Autodesk Inventor part; units mm, degrees
(part 2 of 13)
  line L469 (36.754, 19.2324) -> (36.3194, 18.7979) construction
  line L470 (36.3194, 18.7979) -> (36.3194, 18.2619) construction
  spline S154 degree 3 poles (36.3194, 18.2619) (36.3194, 17.7259) (36.754, 17.2914) (37.29, 17.2914) knots 0 0 0 0 1 1 1 1
  line L471 (36.3194, 18.2619) -> (36.3194, 17.7259) construction
  line L472 (36.3194, 17.7259) -> (36.754, 17.2914) construction
  line L473 (36.754, 17.2914) -> (37.29, 17.2914) construction
  spline S155 degree 3 poles (37.29, 17.2914) (37.826, 17.2914) (38.2606, 17.7259) (38.2606, 18.2619) knots 0 0 0 0 1 1 1 1
  line L474 (37.29, 17.2914) -> (37.826, 17.2914) construction
  line L475 (37.826, 17.2914) -> (38.2606, 17.7259) construction
  line L476 (38.2606, 17.7259) -> (38.2606, 18.2619) construction
  spline S156 degree 3 poles (35.7064, 20.816) (35.7064, 21.352) (35.2719, 21.7866) (34.7358, 21.7866) knots 0 0 0 0 1 1 1 1
  line L477 (35.7064, 20.816) -> (35.7064, 21.352) construction
  line L478 (35.7064, 21.352) -> (35.2719, 21.7866) construction
  line L479 (35.2719, 21.7866) -> (34.7358, 21.7866) construction
  spline S157 degree 3 poles (34.7358, 21.7866) (34.1999, 21.7866) (33.7653, 21.352) (33.7653, 20.816) knots 0 0 0 0 1 1 1 1
  line L480 (34.7358, 21.7866) -> (34.1999, 21.7866) construction
  line L481 (34.1999, 21.7866) -> (33.7653, 21.352) construction
  line L482 (33.7653, 21.352) -> (33.7653, 20.816) construction
  spline S158 degree 3 poles (33.7653, 20.816) (33.7653, 20.28) (34.1999, 19.8455) (34.7358, 19.8455) knots 0 0 0 0 1 1 1 1
  line L483 (33.7653, 20.816) -> (33.7653, 20.28) construction
  line L484 (33.7653, 20.28) -> (34.1999, 19.8455) construction
  line L485 (34.1999, 19.8455) -> (34.7358, 19.8455) construction
  spline S159 degree 3 poles (34.7358, 19.8455) (35.2719, 19.8455) (35.7064, 20.28) (35.7064, 20.816) knots 0 0 0 0 1 1 1 1
  line L486 (34.7358, 19.8455) -> (35.2719, 19.8455) construction
  line L487 (35.2719, 19.8455) -> (35.7064, 20.28) construction
  line L488 (35.7064, 20.28) -> (35.7064, 20.816) construction
  spline S160 degree 3 poles (35.7064, 23.3701) (35.7064, 23.9061) (35.2719, 24.3407) (34.7358, 24.3407) knots 0 0 0 0 1 1 1 1
  line L489 (35.7064, 23.3701) -> (35.7064, 23.9061) construction
  line L490 (35.7064, 23.9061) -> (35.2719, 24.3407) construction
  line L491 (35.2719, 24.3407) -> (34.7358, 24.3407) construction
  spline S161 degree 3 poles (34.7358, 24.3407) (34.1999, 24.3407) (33.7653, 23.9061) (33.7653, 23.3701) knots 0 0 0 0 1 1 1 1
  line L492 (34.7358, 24.3407) -> (34.1999, 24.3407) construction
  line L493 (34.1999, 24.3407) -> (33.7653, 23.9061) construction
  line L494 (33.7653, 23.9061) -> (33.7653, 23.3701) construction
  spline S162 degree 3 poles (33.7653, 23.3701) (33.7653, 22.8341) (34.1999, 22.3996) (34.7358, 22.3996) knots 0 0 0 0 1 1 1 1
  line L495 (33.7653, 23.3701) -> (33.7653, 22.8341) construction
  line L496 (33.7653, 22.8341) -> (34.1999, 22.3996) construction
  line L497 (34.1999, 22.3996) -> (34.7358, 22.3996) construction
  spline S163 degree 3 poles (34.7358, 22.3996) (35.2719, 22.3996) (35.7064, 22.8341) (35.7064, 23.3701) knots 0 0 0 0 1 1 1 1
  line L498 (34.7358, 22.3996) -> (35.2719, 22.3996) construction
  line L499 (35.2719, 22.3996) -> (35.7064, 22.8341) construction
  line L500 (35.7064, 22.8341) -> (35.7064, 23.3701) construction
  spline S164 degree 3 poles (35.7064, 25.9242) (35.7064, 26.4602) (35.2719, 26.8948) (34.7358, 26.8948) knots 0 0 0 0 1 1 1 1
  line L501 (35.7064, 25.9242) -> (35.7064, 26.4602) construction
  line L502 (35.7064, 26.4602) -> (35.2719, 26.8948) construction
  line L503 (35.2719, 26.8948) -> (34.7358, 26.8948) construction
  spline S165 degree 3 poles (34.7358, 26.8948) (34.1999, 26.8948) (33.7653, 26.4602) (33.7653, 25.9242) knots 0 0 0 0 1 1 1 1
  line L504 (34.7358, 26.8948) -> (34.1999, 26.8948) construction
  line L505 (34.1999, 26.8948) -> (33.7653, 26.4602) construction
  line L506 (33.7653, 26.4602) -> (33.7653, 25.9242) construction
  spline S166 degree 3 poles (33.7653, 25.9242) (33.7653, 25.3882) (34.1999, 24.9537) (34.7358, 24.9537) knots 0 0 0 0 1 1 1 1
  line L507 (33.7653, 25.9242) -> (33.7653, 25.3882) construction
  line L508 (33.7653, 25.3882) -> (34.1999, 24.9537) construction
  line L509 (34.1999, 24.9537) -> (34.7358, 24.9537) construction
  spline S167 degree 3 poles (34.7358, 24.9537) (35.2719, 24.9537) (35.7064, 25.3882) (35.7064, 25.9242) knots 0 0 0 0 1 1 1 1
  line L510 (34.7358, 24.9537) -> (35.2719, 24.9537) construction
  line L511 (35.2719, 24.9537) -> (35.7064, 25.3882) construction
  line L512 (35.7064, 25.3882) -> (35.7064, 25.9242) construction
  spline S168 degree 3 poles (35.7064, 28.4784) (35.7064, 29.0143) (35.2719, 29.4489) (34.7358, 29.4489) knots 0 0 0 0 1 1 1 1
  line L513 (35.7064, 28.4784) -> (35.7064, 29.0143) construction
  line L514 (35.7064, 29.0143) -> (35.2719, 29.4489) construction
  line L515 (35.2719, 29.4489) -> (34.7358, 29.4489) construction
  spline S169 degree 3 poles (34.7358, 29.4489) (34.1999, 29.4489) (33.7653, 29.0143) (33.7653, 28.4784) knots 0 0 0 0 1 1 1 1
  line L516 (34.7358, 29.4489) -> (34.1999, 29.4489) construction
  line L517 (34.1999, 29.4489) -> (33.7653, 29.0143) construction
  line L518 (33.7653, 29.0143) -> (33.7653, 28.4784) construction
  spline S170 degree 3 poles (33.7653, 28.4784) (33.7653, 27.9423) (34.1999, 27.5078) (34.7358, 27.5078) knots 0 0 0 0 1 1 1 1
  line L519 (33.7653, 28.4784) -> (33.7653, 27.9423) construction
  line L520 (33.7653, 27.9423) -> (34.1999, 27.5078) construction
  line L521 (34.1999, 27.5078) -> (34.7358, 27.5078) construction
  spline S171 degree 3 poles (34.7358, 27.5078) (35.2719, 27.5078) (35.7064, 27.9423) (35.7064, 28.4784) knots 0 0 0 0 1 1 1 1
  line L522 (34.7358, 27.5078) -> (35.2719, 27.5078) construction
  line L523 (35.2719, 27.5078) -> (35.7064, 27.9423) construction
  line L524 (35.7064, 27.9423) -> (35.7064, 28.4784) construction
  spline S172 degree 3 poles (35.7064, 31.0325) (35.7064, 31.5684) (35.2719, 32.003) (34.7358, 32.003) knots 0 0 0 0 1 1 1 1
  line L525 (35.7064, 31.0325) -> (35.7064, 31.5684) construction
  line L526 (35.7064, 31.5684) -> (35.2719, 32.003) construction
  line L527 (35.2719, 32.003) -> (34.7358, 32.003) construction
  spline S173 degree 3 poles (34.7358, 32.003) (34.1999, 32.003) (33.7653, 31.5684) (33.7653, 31.0325) knots 0 0 0 0 1 1 1 1
  line L528 (34.7358, 32.003) -> (34.1999, 32.003) construction
  line L529 (34.1999, 32.003) -> (33.7653, 31.5684) construction
  line L530 (33.7653, 31.5684) -> (33.7653, 31.0325) construction
  spline S174 degree 3 poles (33.7653, 31.0325) (33.7653, 30.4965) (34.1999, 30.0619) (34.7358, 30.0619) knots 0 0 0 0 1 1 1 1
  line L531 (33.7653, 31.0325) -> (33.7653, 30.4965) construction
  line L532 (33.7653, 30.4965) -> (34.1999, 30.0619) construction
  line L533 (34.1999, 30.0619) -> (34.7358, 30.0619) construction
  spline S175 degree 3 poles (34.7358, 30.0619) (35.2719, 30.0619) (35.7064, 30.4965) (35.7064, 31.0325) knots 0 0 0 0 1 1 1 1
  line L534 (34.7358, 30.0619) -> (35.2719, 30.0619) construction
  line L535 (35.2719, 30.0619) -> (35.7064, 30.4965) construction
  line L536 (35.7064, 30.4965) -> (35.7064, 31.0325) construction
  spline S176 degree 3 poles (38.2606, 20.816) (38.2606, 21.352) (37.826, 21.7866) (37.29, 21.7866) knots 0 0 0 0 1 1 1 1
  line L537 (38.2606, 20.816) -> (38.2606, 21.352) construction
  line L538 (38.2606, 21.352) -> (37.826, 21.7866) construction
  line L539 (37.826, 21.7866) -> (37.29, 21.7866) construction
  spline S177 degree 3 poles (37.29, 21.7866) (36.754, 21.7866) (36.3194, 21.352) (36.3194, 20.816) knots 0 0 0 0 1 1 1 1
  line L540 (37.29, 21.7866) -> (36.754, 21.7866) construction
  line L541 (36.754, 21.7866) -> (36.3194, 21.352) construction
  line L542 (36.3194, 21.352) -> (36.3194, 20.816) construction
  spline S178 degree 3 poles (36.3194, 20.816) (36.3194, 20.28) (36.754, 19.8455) (37.29, 19.8455) knots 0 0 0 0 1 1 1 1
  line L543 (36.3194, 20.816) -> (36.3194, 20.28) construction
  line L544 (36.3194, 20.28) -> (36.754, 19.8455) construction
  line L545 (36.754, 19.8455) -> (37.29, 19.8455) construction
  spline S179 degree 3 poles (37.29, 19.8455) (37.826, 19.8455) (38.2606, 20.28) (38.2606, 20.816) knots 0 0 0 0 1 1 1 1
  line L546 (37.29, 19.8455) -> (37.826, 19.8455) construction
  line L547 (37.826, 19.8455) -> (38.2606, 20.28) construction
  line L548 (38.2606, 20.28) -> (38.2606, 20.816) construction
  spline S180 degree 3 poles (38.2606, 23.3701) (38.2606, 23.9061) (37.826, 24.3407) (37.29, 24.3407) knots 0 0 0 0 1 1 1 1
  line L549 (38.2606, 23.3701) -> (38.2606, 23.9061) construction
  line L550 (38.2606, 23.9061) -> (37.826, 24.3407) construction
  line L551 (37.826, 24.3407) -> (37.29, 24.3407) construction
  spline S181 degree 3 poles (37.29, 24.3407) (36.754, 24.3407) (36.3194, 23.9061) (36.3194, 23.3701) knots 0 0 0 0 1 1 1 1
  line L552 (37.29, 24.3407) -> (36.754, 24.3407) construction
  line L553 (36.754, 24.3407) -> (36.3194, 23.9061) construction
  line L554 (36.3194, 23.9061) -> (36.3194, 23.3701) construction
  spline S182 degree 3 poles (36.3194, 23.3701) (36.3194, 22.8341) (36.754, 22.3996) (37.29, 22.3996) knots 0 0 0 0 1 1 1 1
  line L555 (36.3194, 23.3701) -> (36.3194, 22.8341) construction
  line L556 (36.3194, 22.8341) -> (36.754, 22.3996) construction
  line L557 (36.754, 22.3996) -> (37.29, 22.3996) construction
  spline S183 degree 3 poles (37.29, 22.3996) (37.826, 22.3996) (38.2606, 22.8341) (38.2606, 23.3701) knots 0 0 0 0 1 1 1 1
  line L558 (37.29, 22.3996) -> (37.826, 22.3996) construction
  line L559 (37.826, 22.3996) -> (38.2606, 22.8341) construction
  line L560 (38.2606, 22.8341) -> (38.2606, 23.3701) construction
  spline S184 degree 3 poles (38.2606, 25.9242) (38.2606, 26.4602) (37.826, 26.8948) (37.29, 26.8948) knots 0 0 0 0 1 1 1 1
  line L561 (38.2606, 25.9242) -> (38.2606, 26.4602) construction
  line L562 (38.2606, 26.4602) -> (37.826, 26.8948) construction
  line L563 (37.826, 26.8948) -> (37.29, 26.8948) construction
  spline S185 degree 3 poles (37.29, 26.8948) (36.754, 26.8948) (36.3194, 26.4602) (36.3194, 25.9242) knots 0 0 0 0 1 1 1 1
  line L564 (37.29, 26.8948) -> (36.754, 26.8948) construction
  line L565 (36.754, 26.8948) -> (36.3194, 26.4602) construction
  line L566 (36.3194, 26.4602) -> (36.3194, 25.9242) construction
  spline S186 degree 3 poles (36.3194, 25.9242) (36.3194, 25.3882) (36.754, 24.9537) (37.29, 24.9537) knots 0 0 0 0 1 1 1 1
  line L567 (36.3194, 25.9242) -> (36.3194, 25.3882) construction
  line L568 (36.3194, 25.3882) -> (36.754, 24.9537) construction
  line L569 (36.754, 24.9537) -> (37.29, 24.9537) construction
  spline S187 degree 3 poles (37.29, 24.9537) (37.826, 24.9537) (38.2606, 25.3882) (38.2606, 25.9242) knots 0 0 0 0 1 1 1 1
  line L570 (37.29, 24.9537) -> (37.826, 24.9537) construction
  line L571 (37.826, 24.9537) -> (38.2606, 25.3882) construction
  line L572 (38.2606, 25.3882) -> (38.2606, 25.9242) construction
  spline S188 degree 3 poles (38.2606, 28.4784) (38.2606, 29.0143) (37.826, 29.4489) (37.29, 29.4489) knots 0 0 0 0 1 1 1 1
  line L573 (38.2606, 28.4784) -> (38.2606, 29.0143) construction
  line L574 (38.2606, 29.0143) -> (37.826, 29.4489) construction
  line L575 (37.826, 29.4489) -> (37.29, 29.4489) construction
  spline S189 degree 3 poles (37.29, 29.4489) (36.754, 29.4489) (36.3194, 29.0143) (36.3194, 28.4784) knots 0 0 0 0 1 1 1 1
  line L576 (37.29, 29.4489) -> (36.754, 29.4489) construction
  line L577 (36.754, 29.4489) -> (36.3194, 29.0143) construction
  line L578 (36.3194, 29.0143) -> (36.3194, 28.4784) construction
  spline S190 degree 3 poles (36.3194, 28.4784) (36.3194, 27.9423) (36.754, 27.5078) (37.29, 27.5078) knots 0 0 0 0 1 1 1 1
  line L579 (36.3194, 28.4784) -> (36.3194, 27.9423) construction
  line L580 (36.3194, 27.9423) -> (36.754, 27.5078) construction
  line L581 (36.754, 27.5078) -> (37.29, 27.5078) construction
  spline S191 degree 3 poles (37.29, 27.5078) (37.826, 27.5078) (38.2606, 27.9423) (38.2606, 28.4784) knots 0 0 0 0 1 1 1 1
  line L582 (37.29, 27.5078) -> (37.826, 27.5078) construction
  line L583 (37.826, 27.5078) -> (38.2606, 27.9423) construction
  line L584 (38.2606, 27.9423) -> (38.2606, 28.4784) construction
  spline S192 degree 3 poles (38.2606, 31.0325) (38.2606, 31.5684) (37.826, 32.003) (37.29, 32.003) knots 0 0 0 0 1 1 1 1
  line L585 (38.2606, 31.0325) -> (38.2606, 31.5684) construction
  line L586 (38.2606, 31.5684) -> (37.826, 32.003) construction
  line L587 (37.826, 32.003) -> (37.29, 32.003) construction
  spline S193 degree 3 poles (37.29, 32.003) (36.754, 32.003) (36.3194, 31.5684) (36.3194, 31.0325) knots 0 0 0 0 1 1 1 1
  line L588 (37.29, 32.003) -> (36.754, 32.003) construction
  line L589 (36.754, 32.003) -> (36.3194, 31.5684) construction
  line L590 (36.3194, 31.5684) -> (36.3194, 31.0325) construction
  spline S194 degree 3 poles (36.3194, 31.0325) (36.3194, 30.4965) (36.754, 30.0619) (37.29, 30.0619) knots 0 0 0 0 1 1 1 1
  line L591 (36.3194, 31.0325) -> (36.3194, 30.4965) construction
  line L592 (36.3194, 30.4965) -> (36.754, 30.0619) construction
  line L593 (36.754, 30.0619) -> (37.29, 30.0619) construction
  spline S195 degree 3 poles (37.29, 30.0619) (37.826, 30.0619) (38.2606, 30.4965) (38.2606, 31.0325) knots 0 0 0 0 1 1 1 1
  line L594 (37.29, 30.0619) -> (37.826, 30.0619) construction
  line L595 (37.826, 30.0619) -> (38.2606, 30.4965) construction
  line L596 (38.2606, 30.4965) -> (38.2606, 31.0325) construction
  spline S196 degree 3 poles (45.9229, 0.3832) (45.9229, 0.9191) (45.4883, 1.3537) (44.9523, 1.3537) knots 0 0 0 0 1 1 1 1
  line L597 (45.9229, 0.3832) -> (45.9229, 0.9191) construction
  line L598 (45.9229, 0.9191) -> (45.4883, 1.3537) construction
  line L599 (45.4883, 1.3537) -> (44.9523, 1.3537) construction
  spline S197 degree 3 poles (44.9523, 1.3537) (44.4163, 1.3537) (43.9818, 0.9191) (43.9818, 0.3832) knots 0 0 0 0 1 1 1 1
  line L600 (44.9523, 1.3537) -> (44.4163, 1.3537) construction
  line L601 (44.4163, 1.3537) -> (43.9818, 0.9191) construction
  line L602 (43.9818, 0.9191) -> (43.9818, 0.3832) construction
  spline S198 degree 3 poles (43.9818, 0.3832) (43.9818, -0.1529) (44.4163, -0.5874) (44.9523, -0.5874) knots 0 0 0 0 1 1 1 1
  line L603 (43.9818, 0.3832) -> (43.9818, -0.1529) construction
  line L604 (43.9818, -0.1529) -> (44.4163, -0.5874) construction
  line L605 (44.4163, -0.5874) -> (44.9523, -0.5874) construction
  spline S199 degree 3 poles (44.9523, -0.5874) (45.4883, -0.5874) (45.9229, -0.1529) (45.9229, 0.3832) knots 0 0 0 0 1 1 1 1
  line L606 (44.9523, -0.5874) -> (45.4883, -0.5874) construction
  line L607 (45.4883, -0.5874) -> (45.9229, -0.1529) construction
  line L608 (45.9229, -0.1529) -> (45.9229, 0.3832) construction
  spline S200 degree 3 poles (48.477, 0.3832) (48.477, 0.9191) (48.0424, 1.3537) (47.5064, 1.3537) knots 0 0 0 0 1 1 1 1
  line L609 (48.477, 0.3832) -> (48.477, 0.9191) construction
  line L610 (48.477, 0.9191) -> (48.0424, 1.3537) construction
  line L611 (48.0424, 1.3537) -> (47.5064, 1.3537) construction
  spline S201 degree 3 poles (47.5064, 1.3537) (46.9704, 1.3537) (46.5359, 0.9191) (46.5359, 0.3832) knots 0 0 0 0 1 1 1 1
  line L612 (47.5064, 1.3537) -> (46.9704, 1.3537) construction
  line L613 (46.9704, 1.3537) -> (46.5359, 0.9191) construction
  line L614 (46.5359, 0.9191) -> (46.5359, 0.3832) construction
  spline S202 degree 3 poles (46.5359, 0.3832) (46.5359, -0.1529) (46.9704, -0.5874) (47.5064, -0.5874) knots 0 0 0 0 1 1 1 1
  line L615 (46.5359, 0.3832) -> (46.5359, -0.1529) construction
  line L616 (46.5359, -0.1529) -> (46.9704, -0.5874) construction
  line L617 (46.9704, -0.5874) -> (47.5064, -0.5874) construction
  spline S203 degree 3 poles (47.5064, -0.5874) (48.0424, -0.5874) (48.477, -0.1529) (48.477, 0.3832) knots 0 0 0 0 1 1 1 1
  line L618 (47.5064, -0.5874) -> (48.0424, -0.5874) construction
  line L619 (48.0424, -0.5874) -> (48.477, -0.1529) construction
  line L620 (48.477, -0.1529) -> (48.477, 0.3832) construction
  spline S204 degree 3 poles (47.3149, 9.7057) (47.3149, 10.9399) (46.3142, 11.9405) (45.08, 11.9405) knots 0 0 0 0 1 1 1 1
  line L621 (47.3149, 9.7057) -> (47.3149, 10.9399) construction
  line L622 (47.3149, 10.9399) -> (46.3142, 11.9405) construction
  line L623 (46.3142, 11.9405) -> (45.08, 11.9405) construction
  spline S205 degree 3 poles (45.08, 11.9405) (43.8459, 11.9405) (42.8452, 10.9399) (42.8452, 9.7057) knots 0 0 0 0 1 1 1 1
  line L624 (45.08, 11.9405) -> (43.8459, 11.9405) construction
  line L625 (43.8459, 11.9405) -> (42.8452, 10.9399) construction
  line L626 (42.8452, 10.9399) -> (42.8452, 9.7057) construction
  spline S206 degree 3 poles (42.8452, 9.7057) (42.8452, 8.4714) (43.8459, 7.4708) (45.08, 7.4708) knots 0 0 0 0 1 1 1 1
  line L627 (42.8452, 9.7057) -> (42.8452, 8.4714) construction
  line L628 (42.8452, 8.4714) -> (43.8459, 7.4708) construction
  line L629 (43.8459, 7.4708) -> (45.08, 7.4708) construction
  spline S207 degree 3 poles (45.08, 7.4708) (46.3142, 7.4708) (47.3149, 8.4714) (47.3149, 9.7057) knots 0 0 0 0 1 1 1 1
  line L630 (45.08, 7.4708) -> (46.3142, 7.4708) construction
  line L631 (46.3142, 7.4708) -> (47.3149, 8.4714) construction
  line L632 (47.3149, 8.4714) -> (47.3149, 9.7057) construction
  spline S208 degree 3 poles (53.5724, 9.7057) (53.5724, 10.8694) (52.6292, 11.8128) (51.4653, 11.8128) knots 0 0 0 0 1 1 1 1
  line L633 (53.5724, 9.7057) -> (53.5724, 10.8694) construction
  line L634 (53.5724, 10.8694) -> (52.6292, 11.8128) construction
  line L635 (52.6292, 11.8128) -> (51.4653, 11.8128) construction
  spline S209 degree 3 poles (51.4653, 11.8128) (50.3018, 11.8128) (49.3582, 10.8694) (49.3582, 9.7057) knots 0 0 0 0 1 1 1 1
  line L636 (51.4653, 11.8128) -> (50.3018, 11.8128) construction
  line L637 (50.3018, 11.8128) -> (49.3582, 10.8694) construction
  line L638 (49.3582, 10.8694) -> (49.3582, 9.7057) construction
  spline S210 degree 3 poles (49.3582, 9.7057) (49.3582, 8.542) (50.3018, 7.5984) (51.4653, 7.5984) knots 0 0 0 0 1 1 1 1
  line L639 (49.3582, 9.7057) -> (49.3582, 8.542) construction
  line L640 (49.3582, 8.542) -> (50.3018, 7.5984) construction
  line L641 (50.3018, 7.5984) -> (51.4653, 7.5984) construction
  spline S211 degree 3 poles (51.4653, 7.5984) (52.6292, 7.5984) (53.5724, 8.542) (53.5724, 9.7057) knots 0 0 0 0 1 1 1 1
  line L642 (51.4653, 7.5984) -> (52.6292, 7.5984) construction
  line L643 (52.6292, 7.5984) -> (53.5724, 8.542) construction
  line L644 (53.5724, 8.542) -> (53.5724, 9.7057) construction
  spline S212 degree 3 poles (50.316, 14.303) (50.316, 15.4314) (49.4011, 16.3463) (48.2727, 16.3463) knots 0 0 0 0 1 1 1 1
  line L645 (50.316, 14.303) -> (50.316, 15.4314) construction
  line L646 (50.316, 15.4314) -> (49.4011, 16.3463) construction
  line L647 (49.4011, 16.3463) -> (48.2727, 16.3463) construction
  spline S213 degree 3 poles (48.2727, 16.3463) (47.1442, 16.3463) (46.2294, 15.4314) (46.2294, 14.303) knots 0 0 0 0 1 1 1 1
  line L648 (48.2727, 16.3463) -> (47.1442, 16.3463) construction
  line L649 (47.1442, 16.3463) -> (46.2294, 15.4314) construction
  line L650 (46.2294, 15.4314) -> (46.2294, 14.303) construction
  spline S214 degree 3 poles (46.2294, 14.303) (46.2294, 13.1746) (47.1442, 12.2598) (48.2727, 12.2598) knots 0 0 0 0 1 1 1 1
  line L651 (46.2294, 14.303) -> (46.2294, 13.1746) construction
  line L652 (46.2294, 13.1746) -> (47.1442, 12.2598) construction
  line L653 (47.1442, 12.2598) -> (48.2727, 12.2598) construction
  spline S215 degree 3 poles (48.2727, 12.2598) (49.4011, 12.2598) (50.316, 13.1746) (50.316, 14.303) knots 0 0 0 0 1 1 1 1
  line L654 (48.2727, 12.2598) -> (49.4011, 12.2598) construction
  line L655 (49.4011, 12.2598) -> (50.316, 13.1746) construction
  line L656 (50.316, 13.1746) -> (50.316, 14.303) construction
  spline S216 degree 3 poles (10.1653, 0.3832) (10.1653, 0.9191) (9.7308, 1.3537) (9.1948, 1.3537) knots 0 0 0 0 1 1 1 1
  line L657 (10.1653, 0.3832) -> (10.1653, 0.9191) construction
  line L658 (10.1653, 0.9191) -> (9.7308, 1.3537) construction
  line L659 (9.7308, 1.3537) -> (9.1948, 1.3537) construction
  spline S217 degree 3 poles (9.1948, 1.3537) (8.6588, 1.3537) (8.2242, 0.9191) (8.2242, 0.3832) knots 0 0 0 0 1 1 1 1
  line L660 (9.1948, 1.3537) -> (8.6588, 1.3537) construction
  line L661 (8.6588, 1.3537) -> (8.2242, 0.9191) construction
  line L662 (8.2242, 0.9191) -> (8.2242, 0.3832) construction
  spline S218 degree 3 poles (8.2242, 0.3832) (8.2242, -0.1529) (8.6588, -0.5874) (9.1948, -0.5874) knots 0 0 0 0 1 1 1 1
  line L663 (8.2242, 0.3832) -> (8.2242, -0.1529) construction
  line L664 (8.2242, -0.1529) -> (8.6588, -0.5874) construction
  line L665 (8.6588, -0.5874) -> (9.1948, -0.5874) construction
  spline S219 degree 3 poles (9.1948, -0.5874) (9.7308, -0.5874) (10.1653, -0.1529) (10.1653, 0.3832) knots 0 0 0 0 1 1 1 1
  line L666 (9.1948, -0.5874) -> (9.7308, -0.5874) construction
  line L667 (9.7308, -0.5874) -> (10.1653, -0.1529) construction
  line L668 (10.1653, -0.1529) -> (10.1653, 0.3832) construction
  spline S220 degree 3 poles (12.7194, 0.3832) (12.7194, 0.9191) (12.2849, 1.3537) (11.7489, 1.3537) knots 0 0 0 0 1 1 1 1
  line L669 (12.7194, 0.3832) -> (12.7194, 0.9191) construction
  line L670 (12.7194, 0.9191) -> (12.2849, 1.3537) construction
  line L671 (12.2849, 1.3537) -> (11.7489, 1.3537) construction
  spline S221 degree 3 poles (11.7489, 1.3537) (11.2129, 1.3537) (10.7783, 0.9191) (10.7783, 0.3832) knots 0 0 0 0 1 1 1 1
  line L672 (11.7489, 1.3537) -> (11.2129, 1.3537) construction
  line L673 (11.2129, 1.3537) -> (10.7783, 0.9191) construction
  line L674 (10.7783, 0.9191) -> (10.7783, 0.3832) construction
  spline S222 degree 3 poles (10.7783, 0.3832) (10.7783, -0.1529) (11.2129, -0.5874) (11.7489, -0.5874) knots 0 0 0 0 1 1 1 1
  line L675 (10.7783, 0.3832) -> (10.7783, -0.1529) construction
  line L676 (10.7783, -0.1529) -> (11.2129, -0.5874) construction
  line L677 (11.2129, -0.5874) -> (11.7489, -0.5874) construction
  spline S223 degree 3 poles (11.7489, -0.5874) (12.2849, -0.5874) (12.7194, -0.1529) (12.7194, 0.3832) knots 0 0 0 0 1 1 1 1
  line L678 (11.7489, -0.5874) -> (12.2849, -0.5874) construction
  line L679 (12.2849, -0.5874) -> (12.7194, -0.1529) construction
  line L680 (12.7194, -0.1529) -> (12.7194, 0.3832) construction
  spline S224 degree 3 poles (15.2735, 0.3832) (15.2735, 0.9191) (14.839, 1.3537) (14.303, 1.3537) knots 0 0 0 0 1 1 1 1
  line L681 (15.2735, 0.3832) -> (15.2735, 0.9191) construction
  line L682 (15.2735, 0.9191) -> (14.839, 1.3537) construction
  line L683 (14.839, 1.3537) -> (14.303, 1.3537) construction
  spline S225 degree 3 poles (14.303, 1.3537) (13.767, 1.3537) (13.3324, 0.9191) (13.3324, 0.3832) knots 0 0 0 0 1 1 1 1
  line L684 (14.303, 1.3537) -> (13.767, 1.3537) construction
  line L685 (13.767, 1.3537) -> (13.3324, 0.9191) construction
  line L686 (13.3324, 0.9191) -> (13.3324, 0.3832) construction
  spline S226 degree 3 poles (13.3324, 0.3832) (13.3324, -0.1529) (13.767, -0.5874) (14.303, -0.5874) knots 0 0 0 0 1 1 1 1
  line L687 (13.3324, 0.3832) -> (13.3324, -0.1529) construction
  line L688 (13.3324, -0.1529) -> (13.767, -0.5874) construction
  line L689 (13.767, -0.5874) -> (14.303, -0.5874) construction
  spline S227 degree 3 poles (14.303, -0.5874) (14.839, -0.5874) (15.2735, -0.1529) (15.2735, 0.3832) knots 0 0 0 0 1 1 1 1
  line L690 (14.303, -0.5874) -> (14.839, -0.5874) construction
  line L691 (14.839, -0.5874) -> (15.2735, -0.1529) construction
  line L692 (15.2735, -0.1529) -> (15.2735, 0.3832) construction
  spline S228 degree 3 poles (17.8276, 0.3832) (17.8276, 0.9191) (17.3931, 1.3537) (16.8571, 1.3537) knots 0 0 0 0 1 1 1 1
  line L693 (17.8276, 0.3832) -> (17.8276, 0.9191) construction
  line L694 (17.8276, 0.9191) -> (17.3931, 1.3537) construction
  line L695 (17.3931, 1.3537) -> (16.8571, 1.3537) construction
  spline S229 degree 3 poles (16.8571, 1.3537) (16.3211, 1.3537) (15.8866, 0.9191) (15.8866, 0.3832) knots 0 0 0 0 1 1 1 1
  line L696 (16.8571, 1.3537) -> (16.3211, 1.3537) construction
  line L697 (16.3211, 1.3537) -> (15.8866, 0.9191) construction
  line L698 (15.8866, 0.9191) -> (15.8866, 0.3832) construction
  spline S230 degree 3 poles (15.8866, 0.3832) (15.8866, -0.1529) (16.3211, -0.5874) (16.8571, -0.5874) knots 0 0 0 0 1 1 1 1
  line L699 (15.8866, 0.3832) -> (15.8866, -0.1529) construction
  line L700 (15.8866, -0.1529) -> (16.3211, -0.5874) construction
  line L701 (16.3211, -0.5874) -> (16.8571, -0.5874) construction
  spline S231 degree 3 poles (16.8571, -0.5874) (17.3931, -0.5874) (17.8276, -0.1529) (17.8276, 0.3832) knots 0 0 0 0 1 1 1 1
  line L702 (16.8571, -0.5874) -> (17.3931, -0.5874) construction
  line L703 (17.3931, -0.5874) -> (17.8276, -0.1529) construction
  line L704 (17.8276, -0.1529) -> (17.8276, 0.3832) construction
  spline S232 degree 3 poles (17.8276, 2.9373) (17.8276, 3.4732) (17.3931, 3.9078) (16.8571, 3.9078) knots 0 0 0 0 1 1 1 1
  line L705 (17.8276, 2.9373) -> (17.8276, 3.4732) construction
  line L706 (17.8276, 3.4732) -> (17.3931, 3.9078) construction
  line L707 (17.3931, 3.9078) -> (16.8571, 3.9078) construction
  spline S233 degree 3 poles (16.8571, 3.9078) (16.3211, 3.9078) (15.8866, 3.4732) (15.8866, 2.9373) knots 0 0 0 0 1 1 1 1
  line L708 (16.8571, 3.9078) -> (16.3211, 3.9078) construction
  line L709 (16.3211, 3.9078) -> (15.8866, 3.4732) construction
  line L710 (15.8866, 3.4732) -> (15.8866, 2.9373) construction
  spline S234 degree 3 poles (15.8866, 2.9373) (15.8866, 2.4013) (16.3211, 1.9667) (16.8571, 1.9667) knots 0 0 0 0 1 1 1 1
  line L711 (15.8866, 2.9373) -> (15.8866, 2.4013) construction
  line L712 (15.8866, 2.4013) -> (16.3211, 1.9667) construction
  line L713 (16.3211, 1.9667) -> (16.8571, 1.9667) construction
  spline S235 degree 3 poles (16.8571, 1.9667) (17.3931, 1.9667) (17.8276, 2.4013) (17.8276, 2.9373) knots 0 0 0 0 1 1 1 1
  line L714 (16.8571, 1.9667) -> (17.3931, 1.9667) construction
  line L715 (17.3931, 1.9667) -> (17.8276, 2.4013) construction
  line L716 (17.8276, 2.4013) -> (17.8276, 2.9373) construction
  spline S236 degree 3 poles (20.3818, 2.9373) (20.3818, 3.4732) (19.9472, 3.9078) (19.4112, 3.9078) knots 0 0 0 0 1 1 1 1
  line L717 (20.3818, 2.9373) -> (20.3818, 3.4732) construction
  line L718 (20.3818, 3.4732) -> (19.9472, 3.9078) construction
  line L719 (19.9472, 3.9078) -> (19.4112, 3.9078) construction
  spline S237 degree 3 poles (19.4112, 3.9078) (18.8752, 3.9078) (18.4407, 3.4732) (18.4407, 2.9373) knots 0 0 0 0 1 1 1 1
  line L720 (19.4112, 3.9078) -> (18.8752, 3.9078) construction
  line L721 (18.8752, 3.9078) -> (18.4407, 3.4732) construction
  line L722 (18.4407, 3.4732) -> (18.4407, 2.9373) construction
  spline S238 degree 3 poles (18.4407, 2.9373) (18.4407, 2.4013) (18.8752, 1.9667) (19.4112, 1.9667) knots 0 0 0 0 1 1 1 1
  line L723 (18.4407, 2.9373) -> (18.4407, 2.4013) construction
  line L724 (18.4407, 2.4013) -> (18.8752, 1.9667) construction
  line L725 (18.8752, 1.9667) -> (19.4112, 1.9667) construction
  spline S239 degree 3 poles (19.4112, 1.9667) (19.9472, 1.9667) (20.3818, 2.4013) (20.3818, 2.9373) knots 0 0 0 0 1 1 1 1
  line L726 (19.4112, 1.9667) -> (19.9472, 1.9667) construction
  line L727 (19.9472, 1.9667) -> (20.3818, 2.4013) construction
  line L728 (20.3818, 2.4013) -> (20.3818, 2.9373) construction
  spline S240 degree 3 poles (26.767, 0.3832) (26.767, 0.9191) (26.3325, 1.3537) (25.7965, 1.3537) knots 0 0 0 0 1 1 1 1
  line L729 (26.767, 0.3832) -> (26.767, 0.9191) construction
  line L730 (26.767, 0.9191) -> (26.3325, 1.3537) construction
  line L731 (26.3325, 1.3537) -> (25.7965, 1.3537) construction
  spline S241 degree 3 poles (25.7965, 1.3537) (25.2605, 1.3537) (24.8259, 0.9191) (24.8259, 0.3832) knots 0 0 0 0 1 1 1 1
  line L732 (25.7965, 1.3537) -> (25.2605, 1.3537) construction
  line L733 (25.2605, 1.3537) -> (24.8259, 0.9191) construction
  line L734 (24.8259, 0.9191) -> (24.8259, 0.3832) construction
  spline S242 degree 3 poles (24.8259, 0.3832) (24.8259, -0.1529) (25.2605, -0.5874) (25.7965, -0.5874) knots 0 0 0 0 1 1 1 1
  line L735 (24.8259, 0.3832) -> (24.8259, -0.1529) construction
  line L736 (24.8259, -0.1529) -> (25.2605, -0.5874) construction
  line L737 (25.2605, -0.5874) -> (25.7965, -0.5874) construction
  spline S243 degree 3 poles (25.7965, -0.5874) (26.3325, -0.5874) (26.767, -0.1529) (26.767, 0.3832) knots 0 0 0 0 1 1 1 1
  line L738 (25.7965, -0.5874) -> (26.3325, -0.5874) construction
  line L739 (26.3325, -0.5874) -> (26.767, -0.1529) construction
  line L740 (26.767, -0.1529) -> (26.767, 0.3832) construction
  spline S244 degree 3 poles (24.2129, 0.3832) (24.2129, 0.9191) (23.7784, 1.3537) (23.2424, 1.3537) knots 0 0 0 0 1 1 1 1
  line L741 (24.2129, 0.3832) -> (24.2129, 0.9191) construction
  line L742 (24.2129, 0.9191) -> (23.7784, 1.3537) construction
  line L743 (23.7784, 1.3537) -> (23.2424, 1.3537) construction
  spline S245 degree 3 poles (23.2424, 1.3537) (22.7064, 1.3537) (22.2718, 0.9191) (22.2718, 0.3832) knots 0 0 0 0 1 1 1 1
  line L744 (23.2424, 1.3537) -> (22.7064, 1.3537) construction
  line L745 (22.7064, 1.3537) -> (22.2718, 0.9191) construction
  line L746 (22.2718, 0.9191) -> (22.2718, 0.3832) construction
  spline S246 degree 3 poles (22.2718, 0.3832) (22.2718, -0.1529) (22.7064, -0.5874) (23.2424, -0.5874) knots 0 0 0 0 1 1 1 1
  line L747 (22.2718, 0.3832) -> (22.2718, -0.1529) construction
  line L748 (22.2718, -0.1529) -> (22.7064, -0.5874) construction
  line L749 (22.7064, -0.5874) -> (23.2424, -0.5874) construction
  spline S247 degree 3 poles (23.2424, -0.5874) (23.7784, -0.5874) (24.2129, -0.1529) (24.2129, 0.3832) knots 0 0 0 0 1 1 1 1
  line L750 (23.2424, -0.5874) -> (23.7784, -0.5874) construction
  line L751 (23.7784, -0.5874) -> (24.2129, -0.1529) construction
  line L752 (24.2129, -0.1529) -> (24.2129, 0.3832) construction
  spline S248 degree 3 poles (21.6588, 0.3832) (21.6588, 0.9191) (21.2243, 1.3537) (20.6882, 1.3537) knots 0 0 0 0 1 1 1 1
  line L753 (21.6588, 0.3832) -> (21.6588, 0.9191) construction
  line L754 (21.6588, 0.9191) -> (21.2243, 1.3537) construction
  line L755 (21.2243, 1.3537) -> (20.6882, 1.3537) construction
  spline S249 degree 3 poles (20.6882, 1.3537) (20.1523, 1.3537) (19.7177, 0.9191) (19.7177, 0.3832) knots 0 0 0 0 1 1 1 1
  line L756 (20.6882, 1.3537) -> (20.1523, 1.3537) construction
  line L757 (20.1523, 1.3537) -> (19.7177, 0.9191) construction
  line L758 (19.7177, 0.9191) -> (19.7177, 0.3832) construction
  spline S250 degree 3 poles (19.7177, 0.3832) (19.7177, -0.1529) (20.1523, -0.5874) (20.6882, -0.5874) knots 0 0 0 0 1 1 1 1
  line L759 (19.7177, 0.3832) -> (19.7177, -0.1529) construction
  line L760 (19.7177, -0.1529) -> (20.1523, -0.5874) construction
  line L761 (20.1523, -0.5874) -> (20.6882, -0.5874) construction
  spline S251 degree 3 poles (20.6882, -0.5874) (21.2243, -0.5874) (21.6588, -0.1529) (21.6588, 0.3832) knots 0 0 0 0 1 1 1 1
  line L762 (20.6882, -0.5874) -> (21.2243, -0.5874) construction
  line L763 (21.2243, -0.5874) -> (21.6588, -0.1529) construction
  line L764 (21.6588, -0.1529) -> (21.6588, 0.3832) construction
  spline S252 degree 3 poles (20.3818, 5.4914) (20.3818, 6.0273) (19.9472, 6.4619) (19.4112, 6.4619) knots 0 0 0 0 1 1 1 1
  line L765 (20.3818, 5.4914) -> (20.3818, 6.0273) construction
  line L766 (20.3818, 6.0273) -> (19.9472, 6.4619) construction
  line L767 (19.9472, 6.4619) -> (19.4112, 6.4619) construction
  spline S253 degree 3 poles (19.4112, 6.4619) (18.8752, 6.4619) (18.4407, 6.0273) (18.4407, 5.4914) knots 0 0 0 0 1 1 1 1
  line L768 (19.4112, 6.4619) -> (18.8752, 6.4619) construction
  line L769 (18.8752, 6.4619) -> (18.4407, 6.0273) construction
  line L770 (18.4407, 6.0273) -> (18.4407, 5.4914) construction
  spline S254 degree 3 poles (18.4407, 5.4914) (18.4407, 4.9554) (18.8752, 4.5208) (19.4112, 4.5208) knots 0 0 0 0 1 1 1 1
  line L771 (18.4407, 5.4914) -> (18.4407, 4.9554) construction
  line L772 (18.4407, 4.9554) -> (18.8752, 4.5208) construction
  line L773 (18.8752, 4.5208) -> (19.4112, 4.5208) construction
  spline S255 degree 3 poles (19.4112, 4.5208) (19.9472, 4.5208) (20.3818, 4.9554) (20.3818, 5.4914) knots 0 0 0 0 1 1 1 1
  line L774 (19.4112, 4.5208) -> (19.9472, 4.5208) construction
  line L775 (19.9472, 4.5208) -> (20.3818, 4.9554) construction
  line L776 (20.3818, 4.9554) -> (20.3818, 5.4914) construction
  spline S256 degree 3 poles (20.3818, 8.0455) (20.3818, 8.5815) (19.9472, 9.016) (19.4112, 9.016) knots 0 0 0 0 1 1 1 1
  line L777 (20.3818, 8.0455) -> (20.3818, 8.5815) construction
  line L778 (20.3818, 8.5815) -> (19.9472, 9.016) construction
  line L779 (19.9472, 9.016) -> (19.4112, 9.016) construction
  spline S257 degree 3 poles (19.4112, 9.016) (18.8752, 9.016) (18.4407, 8.5815) (18.4407, 8.0455) knots 0 0 0 0 1 1 1 1
  line L780 (19.4112, 9.016) -> (18.8752, 9.016) construction
  line L781 (18.8752, 9.016) -> (18.4407, 8.5815) construction
  line L782 (18.4407, 8.5815) -> (18.4407, 8.0455) construction
  spline S258 degree 3 poles (18.4407, 8.0455) (18.4407, 7.5095) (18.8752, 7.0749) (19.4112, 7.0749) knots 0 0 0 0 1 1 1 1
  line L783 (18.4407, 8.0455) -> (18.4407, 7.5095) construction
  line L784 (18.4407, 7.5095) -> (18.8752, 7.0749) construction
  line L785 (18.8752, 7.0749) -> (19.4112, 7.0749) construction
  spline S259 degree 3 poles (19.4112, 7.0749) (19.9472, 7.0749) (20.3818, 7.5095) (20.3818, 8.0455) knots 0 0 0 0 1 1 1 1
  line L786 (19.4112, 7.0749) -> (19.9472, 7.0749) construction
  line L787 (19.9472, 7.0749) -> (20.3818, 7.5095) construction
  line L788 (20.3818, 7.5095) -> (20.3818, 8.0455) construction
  spline S260 degree 3 poles (20.3818, 10.5996) (20.3818, 11.1356) (19.9472, 11.5701) (19.4112, 11.5701) knots 0 0 0 0 1 1 1 1
  line L789 (20.3818, 10.5996) -> (20.3818, 11.1356) construction
  line L790 (20.3818, 11.1356) -> (19.9472, 11.5701) construction
  line L791 (19.9472, 11.5701) -> (19.4112, 11.5701) construction
  spline S261 degree 3 poles (19.4112, 11.5701) (18.8752, 11.5701) (18.4407, 11.1356) (18.4407, 10.5996) knots 0 0 0 0 1 1 1 1
  line L792 (19.4112, 11.5701) -> (18.8752, 11.5701) construction
  line L793 (18.8752, 11.5701) -> (18.4407, 11.1356) construction
  line L794 (18.4407, 11.1356) -> (18.4407, 10.5996) construction
  spline S262 degree 3 poles (18.4407, 10.5996) (18.4407, 10.0636) (18.8752, 9.629) (19.4112, 9.629) knots 0 0 0 0 1 1 1 1
  line L795 (18.4407, 10.5996) -> (18.4407, 10.0636) construction
  line L796 (18.4407, 10.0636) -> (18.8752, 9.629) construction
  line L797 (18.8752, 9.629) -> (19.4112, 9.629) construction
  spline S263 degree 3 poles (19.4112, 9.629) (19.9472, 9.629) (20.3818, 10.0636) (20.3818, 10.5996) knots 0 0 0 0 1 1 1 1
  line L798 (19.4112, 9.629) -> (19.9472, 9.629) construction
  line L799 (19.9472, 9.629) -> (20.3818, 10.0636) construction
  line L800 (20.3818, 10.0636) -> (20.3818, 10.5996) construction
  spline S264 degree 3 poles (23.319, 11.7489) (23.319, 12.2849) (22.8844, 12.7194) (22.3485, 12.7194) knots 0 0 0 0 1 1 1 1
  line L801 (23.319, 11.7489) -> (23.319, 12.2849) construction
  line L802 (23.319, 12.2849) -> (22.8844, 12.7194) construction
  line L803 (22.8844, 12.7194) -> (22.3485, 12.7194) construction
  spline S265 degree 3 poles (22.3485, 12.7194) (21.8125, 12.7194) (21.3779, 12.2849) (21.3779, 11.7489) knots 0 0 0 0 1 1 1 1
  line L804 (22.3485, 12.7194) -> (21.8125, 12.7194) construction
  line L805 (21.8125, 12.7194) -> (21.3779, 12.2849) construction
  line L806 (21.3779, 12.2849) -> (21.3779, 11.7489) construction
  spline S266 degree 3 poles (21.3779, 11.7489) (21.3779, 11.2129) (21.8125, 10.7783) (22.3485, 10.7783) knots 0 0 0 0 1 1 1 1
  line L807 (21.3779, 11.7489) -> (21.3779, 11.2129) construction
  line L808 (21.3779, 11.2129) -> (21.8125, 10.7783) construction
  line L809 (21.8125, 10.7783) -> (22.3485, 10.7783) construction
  spline S267 degree 3 poles (22.3485, 10.7783) (22.8844, 10.7783) (23.319, 11.2129) (23.319, 11.7489) knots 0 0 0 0 1 1 1 1
  line L810 (22.3485, 10.7783) -> (22.8844, 10.7783) construction
  line L811 (22.8844, 10.7783) -> (23.319, 11.2129) construction
  line L812 (23.319, 11.2129) -> (23.319, 11.7489) construction
  spline S268 degree 3 poles (25.8731, 11.7489) (25.8731, 12.2849) (25.4385, 12.7194) (24.9026, 12.7194) knots 0 0 0 0 1 1 1 1
  line L813 (25.8731, 11.7489) -> (25.8731, 12.2849) construction
  line L814 (25.8731, 12.2849) -> (25.4385, 12.7194) construction
  line L815 (25.4385, 12.7194) -> (24.9026, 12.7194) construction
  spline S269 degree 3 poles (24.9026, 12.7194) (24.3666, 12.7194) (23.932, 12.2849) (23.932, 11.7489) knots 0 0 0 0 1 1 1 1
  line L816 (24.9026, 12.7194) -> (24.3666, 12.7194) construction
  line L817 (24.3666, 12.7194) -> (23.932, 12.2849) construction
  line L818 (23.932, 12.2849) -> (23.932, 11.7489) construction
  spline S270 degree 3 poles (23.932, 11.7489) (23.932, 11.2129) (24.3666, 10.7783) (24.9026, 10.7783) knots 0 0 0 0 1 1 1 1
  line L819 (23.932, 11.7489) -> (23.932, 11.2129) construction
  line L820 (23.932, 11.2129) -> (24.3666, 10.7783) construction
  line L821 (24.3666, 10.7783) -> (24.9026, 10.7783) construction
  spline S271 degree 3 poles (24.9026, 10.7783) (25.4385, 10.7783) (25.8731, 11.2129) (25.8731, 11.7489) knots 0 0 0 0 1 1 1 1
  line L822 (24.9026, 10.7783) -> (25.4385, 10.7783) construction
  line L823 (25.4385, 10.7783) -> (25.8731, 11.2129) construction
  line L824 (25.8731, 11.2129) -> (25.8731, 11.7489) construction
  spline S272 degree 3 poles (23.319, 14.303) (23.319, 14.839) (22.8844, 15.2735) (22.3485, 15.2735) knots 0 0 0 0 1 1 1 1
  line L825 (23.319, 14.303) -> (23.319, 14.839) construction
  line L826 (23.319, 14.839) -> (22.8844, 15.2735) construction
  line L827 (22.8844, 15.2735) -> (22.3485, 15.2735) construction
  spline S273 degree 3 poles (22.3485, 15.2735) (21.8125, 15.2735) (21.3779, 14.839) (21.3779, 14.303) knots 0 0 0 0 1 1 1 1
  line L828 (22.3485, 15.2735) -> (21.8125, 15.2735) construction
  line L829 (21.8125, 15.2735) -> (21.3779, 14.839) construction
  line L830 (21.3779, 14.839) -> (21.3779, 14.303) construction
  spline S274 degree 3 poles (21.3779, 14.303) (21.3779, 13.767) (21.8125, 13.3324) (22.3485, 13.3324) knots 0 0 0 0 1 1 1 1
  line L831 (21.3779, 14.303) -> (21.3779, 13.767) construction
  line L832 (21.3779, 13.767) -> (21.8125, 13.3324) construction
  line L833 (21.8125, 13.3324) -> (22.3485, 13.3324) construction
  spline S275 degree 3 poles (22.3485, 13.3324) (22.8844, 13.3324) (23.319, 13.767) (23.319, 14.303) knots 0 0 0 0 1 1 1 1
  line L834 (22.3485, 13.3324) -> (22.8844, 13.3324) construction
  line L835 (22.8844, 13.3324) -> (23.319, 13.767) construction
  line L836 (23.319, 13.767) -> (23.319, 14.303) construction
  spline S276 degree 3 poles (25.8731, 14.303) (25.8731, 14.839) (25.4385, 15.2735) (24.9026, 15.2735) knots 0 0 0 0 1 1 1 1
  line L837 (25.8731, 14.303) -> (25.8731, 14.839) construction
  line L838 (25.8731, 14.839) -> (25.4385, 15.2735) construction
  line L839 (25.4385, 15.2735) -> (24.9026, 15.2735) construction
  spline S277 degree 3 poles (24.9026, 15.2735) (24.3666, 15.2735) (23.932, 14.839) (23.932, 14.303) knots 0 0 0 0 1 1 1 1
  line L840 (24.9026, 15.2735) -> (24.3666, 15.2735) construction
  line L841 (24.3666, 15.2735) -> (23.932, 14.839) construction
  line L842 (23.932, 14.839) -> (23.932, 14.303) construction
  spline S278 degree 3 poles (23.932, 14.303) (23.932, 13.767) (24.3666, 13.3324) (24.9026, 13.3324) knots 0 0 0 0 1 1 1 1
  line L843 (23.932, 14.303) -> (23.932, 13.767) construction
  line L844 (23.932, 13.767) -> (24.3666, 13.3324) construction
  line L845 (24.3666, 13.3324) -> (24.9026, 13.3324) construction
  spline S279 degree 3 poles (24.9026, 13.3324) (25.4385, 13.3324) (25.8731, 13.767) (25.8731, 14.303) knots 0 0 0 0 1 1 1 1
  line L846 (24.9026, 13.3324) -> (25.4385, 13.3324) construction
  line L847 (25.4385, 13.3324) -> (25.8731, 13.767) construction
  line L848 (25.8731, 13.767) -> (25.8731, 14.303) construction
  spline S280 degree 3 poles (17.8276, 5.4914) (17.8276, 6.0273) (17.3931, 6.4619) (16.8571, 6.4619) knots 0 0 0 0 1 1 1 1
  line L849 (17.8276, 5.4914) -> (17.8276, 6.0273) construction
  line L850 (17.8276, 6.0273) -> (17.3931, 6.4619) construction
  line L851 (17.3931, 6.4619) -> (16.8571, 6.4619) construction
  spline S281 degree 3 poles (16.8571, 6.4619) (16.3211, 6.4619) (15.8866, 6.0273) (15.8866, 5.4914) knots 0 0 0 0 1 1 1 1
  line L852 (16.8571, 6.4619) -> (16.3211, 6.4619) construction
  line L853 (16.3211, 6.4619) -> (15.8866, 6.0273) construction
  line L854 (15.8866, 6.0273) -> (15.8866, 5.4914) construction
  spline S282 degree 3 poles (15.8866, 5.4914) (15.8866, 4.9554) (16.3211, 4.5208) (16.8571, 4.5208) knots 0 0 0 0 1 1 1 1
  line L855 (15.8866, 5.4914) -> (15.8866, 4.9554) construction
  line L856 (15.8866, 4.9554) -> (16.3211, 4.5208) construction
  line L857 (16.3211, 4.5208) -> (16.8571, 4.5208) construction
  spline S283 degree 3 poles (16.8571, 4.5208) (17.3931, 4.5208) (17.8276, 4.9554) (17.8276, 5.4914) knots 0 0 0 0 1 1 1 1
  line L858 (16.8571, 4.5208) -> (17.3931, 4.5208) construction
  line L859 (17.3931, 4.5208) -> (17.8276, 4.9554) construction
  line L860 (17.8276, 4.9554) -> (17.8276, 5.4914) construction
  spline S284 degree 3 poles (17.8276, 8.0455) (17.8276, 8.5815) (17.3931, 9.016) (16.8571, 9.016) knots 0 0 0 0 1 1 1 1
  line L861 (17.8276, 8.0455) -> (17.8276, 8.5815) construction
  line L862 (17.8276, 8.5815) -> (17.3931, 9.016) construction
  line L863 (17.3931, 9.016) -> (16.8571, 9.016) construction
  spline S285 degree 3 poles (16.8571, 9.016) (16.3211, 9.016) (15.8866, 8.5815) (15.8866, 8.0455) knots 0 0 0 0 1 1 1 1
  line L864 (16.8571, 9.016) -> (16.3211, 9.016) construction
  line L865 (16.3211, 9.016) -> (15.8866, 8.5815) construction
  line L866 (15.8866, 8.5815) -> (15.8866, 8.0455) construction
  spline S286 degree 3 poles (15.8866, 8.0455) (15.8866, 7.5095) (16.3211, 7.0749) (16.8571, 7.0749) knots 0 0 0 0 1 1 1 1
  line L867 (15.8866, 8.0455) -> (15.8866, 7.5095) construction
  line L868 (15.8866, 7.5095) -> (16.3211, 7.0749) construction
  line L869 (16.3211, 7.0749) -> (16.8571, 7.0749) construction
  spline S287 degree 3 poles (16.8571, 7.0749) (17.3931, 7.0749) (17.8276, 7.5095) (17.8276, 8.0455) knots 0 0 0 0 1 1 1 1
  line L870 (16.8571, 7.0749) -> (17.3931, 7.0749) construction
  line L871 (17.3931, 7.0749) -> (17.8276, 7.5095) construction
  line L872 (17.8276, 7.5095) -> (17.8276, 8.0455) construction
  spline S288 degree 3 poles (17.8276, 10.5996) (17.8276, 11.1356) (17.3931, 11.5701) (16.8571, 11.5701) knots 0 0 0 0 1 1 1 1
  line L873 (17.8276, 10.5996) -> (17.8276, 11.1356) construction
  line L874 (17.8276, 11.1356) -> (17.3931, 11.5701) construction
  line L875 (17.3931, 11.5701) -> (16.8571, 11.5701) construction
  spline S289 degree 3 poles (16.8571, 11.5701) (16.3211, 11.5701) (15.8866, 11.1356) (15.8866, 10.5996) knots 0 0 0 0 1 1 1 1
  line L876 (16.8571, 11.5701) -> (16.3211, 11.5701) construction
  line L877 (16.3211, 11.5701) -> (15.8866, 11.1356) construction
  line L878 (15.8866, 11.1356) -> (15.8866, 10.5996) construction
  spline S290 degree 3 poles (15.8866, 10.5996) (15.8866, 10.0636) (16.3211, 9.629) (16.8571, 9.629) knots 0 0 0 0 1 1 1 1
  line L879 (15.8866, 10.5996) -> (15.8866, 10.0636) construction
  line L880 (15.8866, 10.0636) -> (16.3211, 9.629) construction
  line L881 (16.3211, 9.629) -> (16.8571, 9.629) construction
  spline S291 degree 3 poles (16.8571, 9.629) (17.3931, 9.629) (17.8276, 10.0636) (17.8276, 10.5996) knots 0 0 0 0 1 1 1 1
  line L882 (16.8571, 9.629) -> (17.3931, 9.629) construction
  line L883 (17.3931, 9.629) -> (17.8276, 10.0636) construction
  line L884 (17.8276, 10.0636) -> (17.8276, 10.5996) construction
  spline S292 degree 3 poles (17.8276, 13.1537) (17.8276, 13.6897) (17.3931, 14.1242) (16.8571, 14.1242) knots 0 0 0 0 1 1 1 1
  line L885 (17.8276, 13.1537) -> (17.8276, 13.6897) construction
  line L886 (17.8276, 13.6897) -> (17.3931, 14.1242) construction
  line L887 (17.3931, 14.1242) -> (16.8571, 14.1242) construction
  spline S293 degree 3 poles (16.8571, 14.1242) (16.3211, 14.1242) (15.8866, 13.6897) (15.8866, 13.1537) knots 0 0 0 0 1 1 1 1
  line L888 (16.8571, 14.1242) -> (16.3211, 14.1242) construction
  line L889 (16.3211, 14.1242) -> (15.8866, 13.6897) construction
  line L890 (15.8866, 13.6897) -> (15.8866, 13.1537) construction
  spline S294 degree 3 poles (15.8866, 13.1537) (15.8866, 12.6177) (16.3211, 12.1831) (16.8571, 12.1831) knots 0 0 0 0 1 1 1 1
  line L891 (15.8866, 13.1537) -> (15.8866, 12.6177) construction
  line L892 (15.8866, 12.6177) -> (16.3211, 12.1831) construction
  line L893 (16.3211, 12.1831) -> (16.8571, 12.1831) construction
  spline S295 degree 3 poles (16.8571, 12.1831) (17.3931, 12.1831) (17.8276, 12.6177) (17.8276, 13.1537) knots 0 0 0 0 1 1 1 1
  line L894 (16.8571, 12.1831) -> (17.3931, 12.1831) construction
  line L895 (17.3931, 12.1831) -> (17.8276, 12.6177) construction
  line L896 (17.8276, 12.6177) -> (17.8276, 13.1537) construction
  spline S296 degree 3 poles (17.8276, 15.7078) (17.8276, 16.2438) (17.3931, 16.6783) (16.8571, 16.6783) knots 0 0 0 0 1 1 1 1
  line L897 (17.8276, 15.7078) -> (17.8276, 16.2438) construction
  line L898 (17.8276, 16.2438) -> (17.3931, 16.6783) construction
  line L899 (17.3931, 16.6783) -> (16.8571, 16.6783) construction
  spline S297 degree 3 poles (16.8571, 16.6783) (16.3211, 16.6783) (15.8866, 16.2438) (15.8866, 15.7078) knots 0 0 0 0 1 1 1 1
  line L900 (16.8571, 16.6783) -> (16.3211, 16.6783) construction
  line L901 (16.3211, 16.6783) -> (15.8866, 16.2438) construction
  line L902 (15.8866, 16.2438) -> (15.8866, 15.7078) construction
  spline S298 degree 3 poles (15.8866, 15.7078) (15.8866, 15.1718) (16.3211, 14.7372) (16.8571, 14.7372) knots 0 0 0 0 1 1 1 1
  line L903 (15.8866, 15.7078) -> (15.8866, 15.1718) construction
  line L904 (15.8866, 15.1718) -> (16.3211, 14.7372) construction
  line L905 (16.3211, 14.7372) -> (16.8571, 14.7372) construction
  spline S299 degree 3 poles (16.8571, 14.7372) (17.3931, 14.7372) (17.8276, 15.1718) (17.8276, 15.7078) knots 0 0 0 0 1 1 1 1
  line L906 (16.8571, 14.7372) -> (17.3931, 14.7372) construction
  line L907 (17.3931, 14.7372) -> (17.8276, 15.1718) construction
  line L908 (17.8276, 15.1718) -> (17.8276, 15.7078) construction
  spline S300 degree 3 poles (17.8276, 18.2619) (17.8276, 18.7979) (17.3931, 19.2324) (16.8571, 19.2324) knots 0 0 0 0 1 1 1 1
  line L909 (17.8276, 18.2619) -> (17.8276, 18.7979) construction
  line L910 (17.8276, 18.7979) -> (17.3931, 19.2324) construction
  line L911 (17.3931, 19.2324) -> (16.8571, 19.2324) construction
  spline S301 degree 3 poles (16.8571, 19.2324) (16.3211, 19.2324) (15.8866, 18.7979) (15.8866, 18.2619) knots 0 0 0 0 1 1 1 1
  line L912 (16.8571, 19.2324) -> (16.3211, 19.2324) construction
  line L913 (16.3211, 19.2324) -> (15.8866, 18.7979) construction
  line L914 (15.8866, 18.7979) -> (15.8866, 18.2619) construction
  spline S302 degree 3 poles (15.8866, 18.2619) (15.8866, 17.7259) (16.3211, 17.2914) (16.8571, 17.2914) knots 0 0 0 0 1 1 1 1
  line L915 (15.8866, 18.2619) -> (15.8866, 17.7259) construction
  line L916 (15.8866, 17.7259) -> (16.3211, 17.2914) construction
  line L917 (16.3211, 17.2914) -> (16.8571, 17.2914) construction
  spline S303 degree 3 poles (16.8571, 17.2914) (17.3931, 17.2914) (17.8276, 17.7259) (17.8276, 18.2619) knots 0 0 0 0 1 1 1 1
  line L918 (16.8571, 17.2914) -> (17.3931, 17.2914) construction
  line L919 (17.3931, 17.2914) -> (17.8276, 17.7259) construction
  line L920 (17.8276, 17.7259) -> (17.8276, 18.2619) construction
  spline S304 degree 3 poles (17.8276, 20.816) (17.8276, 21.352) (17.3931, 21.7866) (16.8571, 21.7866) knots 0 0 0 0 1 1 1 1
  line L921 (17.8276, 20.816) -> (17.8276, 21.352) construction
  line L922 (17.8276, 21.352) -> (17.3931, 21.7866) construction
  line L923 (17.3931, 21.7866) -> (16.8571, 21.7866) construction
  spline S305 degree 3 poles (16.8571, 21.7866) (16.3211, 21.7866) (15.8866, 21.352) (15.8866, 20.816) knots 0 0 0 0 1 1 1 1
  line L924 (16.8571, 21.7866) -> (16.3211, 21.7866) construction
  line L925 (16.3211, 21.7866) -> (15.8866, 21.352) construction
  line L926 (15.8866, 21.352) -> (15.8866, 20.816) construction
  spline S306 degree 3 poles (15.8866, 20.816) (15.8866, 20.28) (16.3211, 19.8455) (16.8571, 19.8455) knots 0 0 0 0 1 1 1 1
  line L927 (15.8866, 20.816) -> (15.8866, 20.28) construction
  line L928 (15.8866, 20.28) -> (16.3211, 19.8455) construction
  line L929 (16.3211, 19.8455) -> (16.8571, 19.8455) construction
  spline S307 degree 3 poles (16.8571, 19.8455) (17.3931, 19.8455) (17.8276, 20.28) (17.8276, 20.816) knots 0 0 0 0 1 1 1 1
  line L930 (16.8571, 19.8455) -> (17.3931, 19.8455) construction
  line L931 (17.3931, 19.8455) -> (17.8276, 20.28) construction
  line L932 (17.8276, 20.28) -> (17.8276, 20.816) construction
  spline S308 degree 3 poles (20.3818, 13.1537) (20.3818, 13.6897) (19.9472, 14.1242) (19.4112, 14.1242) knots 0 0 0 0 1 1 1 1
  line L933 (20.3818, 13.1537) -> (20.3818, 13.6897) construction
  line L934 (20.3818, 13.6897) -> (19.9472, 14.1242) construction
  line L935 (19.9472, 14.1242) -> (19.4112, 14.1242) construction
  spline S309 degree 3 poles (19.4112, 14.1242) (18.8752, 14.1242) (18.4407, 13.6897) (18.4407, 13.1537) knots 0 0 0 0 1 1 1 1
  line L936 (19.4112, 14.1242) -> (18.8752, 14.1242) construction
  line L937 (18.8752, 14.1242) -> (18.4407, 13.6897) construction
  line L938 (18.4407, 13.6897) -> (18.4407, 13.1537) construction